Autodesk Fusion 360 part; units mm, degrees
(part 9 of 9)
  spline S33 degree 5 poles (15.6903, -6.8774) (15.6984, -6.8822) (15.7144, -6.892) (15.7381, -6.9074) (15.7688, -6.9292) (15.8062, -6.9579) (15.8428, -6.9878) (15.8789, -7.0185) (15.9148, -7.0495) (15.9505, -7.0809) (15.986, -7.1125) (16.0213, -7.1444) (16.0562, -7.1769) (16.0907, -7.2099) (16.1249, -7.2435) (16.1586, -7.2775) (16.1921, -7.3121) (16.2253, -7.3469) (16.2582, -7.3822) (16.2909, -7.4177) (16.3234, -7.4535) (16.3557, -7.4896) (16.3877, -7.526) (16.4194, -7.5628) (16.4509, -7.6) (16.4821, -7.6374) (16.5131, -7.6752) (16.5439, -7.7132) (16.5744, -7.7515) (16.6048, -7.7901) (16.6349, -7.829) (16.6647, -7.8681) (16.6944, -7.9075) (16.7238, -7.9471) (16.7531, -7.987) (16.7821, -8.0272) (16.8109, -8.0676) (16.8394, -8.1083) (16.8678, -8.1492) (16.896, -8.1903) (16.9239, -8.2317) (16.9517, -8.2733) (16.9792, -8.3151) (17.0066, -8.3572) (17.0337, -8.3994) (17.0607, -8.4419) (17.0874, -8.4846) (17.1139, -8.5276) (17.1403, -8.5707) (17.1664, -8.614) (17.1923, -8.6576) (17.2181, -8.7014) (17.2436, -8.7453) (17.269, -8.7895) (17.2941, -8.8338) (17.3191, -8.8784) (17.3438, -8.9231) (17.3684, -8.9681) (17.3928, -9.0132) (17.417, -9.0585) (17.441, -9.104) (17.4648, -9.1497) (17.4884, -9.1956) (17.5118, -9.2417) (17.535, -9.2879) (17.5581, -9.3343) (17.5809, -9.3809) (17.6036, -9.4277) (17.626, -9.4746) (17.6483, -9.5217) (17.6704, -9.569) (17.6879, -9.6069) (17.701, -9.6355) (17.7096, -9.6545) (17.7139, -9.6641) knots 0 0 0 0 0 0 0.01428571 0.02857143 0.04285714 0.05714286 0.07142857 0.08571429 0.1 0.11428571 0.12857143 0.14285714 0.15714286 0.17142857 0.18571429 0.2 0.21428571 0.22857143 0.24285714 0.25714286 0.27142857 0.28571429 0.3 0.31428571 0.32857143 0.34285714 0.35714286 0.37142857 0.38571429 0.4 0.41428571 0.42857143 0.44285714 0.45714286 0.47142857 0.48571429 0.5 0.51428571 0.52857143 0.54285714 0.55714286 0.57142857 0.58571429 0.6 0.61428571 0.62857143 0.64285714 0.65714286 0.67142857 0.68571429 0.7 0.71428571 0.72857143 0.74285714 0.75714286 0.77142857 0.78571429 0.8 0.81428571 0.82857143 0.84285714 0.85714286 0.87142857 0.88571429 0.9 0.91428571 0.92857143 0.94285714 0.95714286 0.97142857 0.98571429 1 1 1 1 1 1
  line L33 (15.6903, -6.8774) -> (15.3748, -6.6893)
  arc A67 (15.0406, -5.4943) -> (15.3748, -6.6893) centre (15.8355, -5.9162) ccw
  arc A68 (15.0406, -5.4943) -> (15.3066, -4.9723) centre (-0.4607, 2.7328) ccw
  arc A69 (16.4698, -4.5402) -> (15.3066, -4.9723) centre (16.1152, -5.3674) ccw
  line L34 (16.4698, -4.5402) -> (16.8074, -4.6849)
  spline S34 degree 5 poles (16.8074, -4.6849) (16.816, -4.6886) (16.8334, -4.6958) (16.8598, -4.7059) (16.8955, -4.7181) (16.9407, -4.7314) (16.9864, -4.7434) (17.0324, -4.7546) (17.0786, -4.7654) (17.125, -4.7759) (17.1714, -4.786) (17.218, -4.7957) (17.2648, -4.8049) (17.3118, -4.8135) (17.359, -4.8213) (17.4064, -4.8286) (17.454, -4.8354) (17.5017, -4.8417) (17.5496, -4.8477) (17.5975, -4.8533) (17.6456, -4.8585) (17.6938, -4.8634) (17.7421, -4.8679) (17.7905, -4.8719) (17.8391, -4.8756) (17.8877, -4.8788) (17.9365, -4.8817) (17.9853, -4.8842) (18.0343, -4.8864) (18.0833, -4.8883) (18.1325, -4.8898) (18.1817, -4.891) (18.231, -4.8918) (18.2803, -4.8923) (18.3298, -4.8925) (18.3794, -4.8924) (18.429, -4.8919) (18.4787, -4.8911) (18.5284, -4.89) (18.5783, -4.8886) (18.6282, -4.887) (18.6781, -4.885) (18.7282, -4.8827) (18.7782, -4.8801) (18.8284, -4.8772) (18.8786, -4.874) (18.9289, -4.8705) (18.9792, -4.8667) (19.0296, -4.8627) (19.08, -4.8584) (19.1305, -4.8537) (19.181, -4.8488) (19.2316, -4.8437) (19.2822, -4.8382) (19.3329, -4.8325) (19.3836, -4.8265) (19.4344, -4.8202) (19.4852, -4.8137) (19.536, -4.8069) (19.5869, -4.7998) (19.6378, -4.7925) (19.6888, -4.7849) (19.7398, -4.777) (19.7908, -4.7689) (19.8418, -4.7605) (19.8929, -4.7519) (19.944, -4.743) (19.9952, -4.7338) (20.0464, -4.7244) (20.0976, -4.7147) (20.1488, -4.7048) (20.1898, -4.6967) (20.2206, -4.6904) (20.2411, -4.6863) (20.2513, -4.6841) knots 0 0 0 0 0 0 0.01428571 0.02857143 0.04285714 0.05714286 0.07142857 0.08571429 0.1 0.11428571 0.12857143 0.14285714 0.15714286 0.17142857 0.18571429 0.2 0.21428571 0.22857143 0.24285714 0.25714286 0.27142857 0.28571429 0.3 0.31428571 0.32857143 0.34285714 0.35714286 0.37142857 0.38571429 0.4 0.41428571 0.42857143 0.44285714 0.45714286 0.47142857 0.48571429 0.5 0.51428571 0.52857143 0.54285714 0.55714286 0.57142857 0.58571429 0.6 0.61428571 0.62857143 0.64285714 0.65714286 0.67142857 0.68571429 0.7 0.71428571 0.72857143 0.74285714 0.75714286 0.77142857 0.78571429 0.8 0.81428571 0.82857143 0.84285714 0.85714286 0.87142857 0.88571429 0.9 0.91428571 0.92857143 0.94285714 0.95714286 0.97142857 0.98571429 1 1 1 1 1 1
  arc A70 (20.2513, -4.6841) -> (20.6552, -3.441) centre (-0.4607, 2.7328) ccw
  spline S35 degree 5 poles (17.8695, -1.4161) (17.8787, -1.4182) (17.897, -1.4226) (17.9242, -1.4299) (17.9602, -1.4411) (18.0046, -1.4569) (18.0487, -1.474) (18.0925, -1.492) (18.1362, -1.5104) (18.1799, -1.5292) (18.2234, -1.5483) (18.2668, -1.5678) (18.3101, -1.5879) (18.3531, -1.6086) (18.3959, -1.63) (18.4386, -1.6519) (18.4811, -1.6744) (18.5234, -1.6974) (18.5656, -1.7207) (18.6077, -1.7443) (18.6497, -1.7683) (18.6915, -1.7927) (18.7332, -1.8175) (18.7748, -1.8427) (18.8162, -1.8683) (18.8575, -1.8942) (18.8986, -1.9206) (18.9396, -1.9472) (18.9805, -1.9742) (19.0213, -2.0016) (19.0619, -2.0292) (19.1024, -2.0572) (19.1428, -2.0855) (19.183, -2.1141) (19.2232, -2.143) (19.2632, -2.1723) (19.303, -2.2018) (19.3428, -2.2316) (19.3824, -2.2618) (19.4219, -2.2922) (19.4613, -2.3229) (19.5005, -2.3539) (19.5397, -2.3851) (19.5786, -2.4167) (19.6175, -2.4485) (19.6563, -2.4806) (19.6949, -2.513) (19.7334, -2.5456) (19.7718, -2.5785) (19.81, -2.6116) (19.8482, -2.645) (19.8862, -2.6787) (19.924, -2.7126) (19.9618, -2.7468) (19.9994, -2.7812) (20.0369, -2.8158) (20.0743, -2.8507) (20.1116, -2.8859) (20.1487, -2.9213) (20.1857, -2.9569) (20.2226, -2.9928) (20.2593, -3.0289) (20.296, -3.0652) (20.3325, -3.1018) (20.3688, -3.1386) (20.4051, -3.1756) (20.4412, -3.2128) (20.4772, -3.2503) (20.5131, -3.288) (20.5488, -3.3259) (20.5844, -3.3641) (20.6128, -3.3947) (20.6341, -3.4179) (20.6482, -3.4333) (20.6552, -3.441) knots 0 0 0 0 0 0 0.01428571 0.02857143 0.04285714 0.05714286 0.07142857 0.08571429 0.1 0.11428571 0.12857143 0.14285714 0.15714286 0.17142857 0.18571429 0.2 0.21428571 0.22857143 0.24285714 0.25714286 0.27142857 0.28571429 0.3 0.31428571 0.32857143 0.34285714 0.35714286 0.37142857 0.38571429 0.4 0.41428571 0.42857143 0.44285714 0.45714286 0.47142857 0.48571429 0.5 0.51428571 0.52857143 0.54285714 0.55714286 0.57142857 0.58571429 0.6 0.61428571 0.62857143 0.64285714 0.65714286 0.67142857 0.68571429 0.7 0.71428571 0.72857143 0.74285714 0.75714286 0.77142857 0.78571429 0.8 0.81428571 0.82857143 0.84285714 0.85714286 0.87142857 0.88571429 0.9 0.91428571 0.92857143 0.94285714 0.95714286 0.97142857 0.98571429 1 1 1 1 1 1
  line L35 (17.8695, -1.4161) -> (17.5113, -1.3347)
  arc A71 (16.8242, -0.3015) -> (17.5113, -1.3347) centre (17.7106, -0.4571) ccw
  arc A72 (16.8242, -0.3015) -> (16.9158, 0.2772) centre (-0.4607, 2.7328) ccw
  arc A73 (17.8886, 1.0476) -> (16.9158, 0.2772) centre (17.807, 0.1513) ccw
  line L36 (17.8886, 1.0476) -> (18.2544, 1.0142)
  spline S36 degree 5 poles (18.2544, 1.0142) (18.2638, 1.0134) (18.2826, 1.0119) (18.3108, 1.0105) (18.3484, 1.01) (18.3956, 1.0112) (18.4427, 1.0139) (18.49, 1.0175) (18.5373, 1.0215) (18.5845, 1.0259) (18.6318, 1.0306) (18.6792, 1.0358) (18.7265, 1.0415) (18.7738, 1.0479) (18.8212, 1.055) (18.8685, 1.0627) (18.9159, 1.071) (18.9632, 1.0797) (19.0106, 1.0888) (19.0579, 1.0983) (19.1053, 1.1082) (19.1526, 1.1184) (19.1999, 1.1291) (19.2472, 1.1402) (19.2945, 1.1517) (19.3418, 1.1637) (19.3891, 1.176) (19.4363, 1.1887) (19.4835, 1.2018) (19.5307, 1.2152) (19.5779, 1.2289) (19.6251, 1.243) (19.6723, 1.2574) (19.7194, 1.2722) (19.7665, 1.2873) (19.8136, 1.3027) (19.8606, 1.3185) (19.9076, 1.3346) (19.9546, 1.351) (20.0016, 1.3677) (20.0485, 1.3848) (20.0954, 1.4021) (20.1423, 1.4198) (20.1891, 1.4377) (20.2359, 1.456) (20.2827, 1.4745) (20.3294, 1.4933) (20.3761, 1.5125) (20.4228, 1.5319) (20.4694, 1.5516) (20.516, 1.5716) (20.5625, 1.5919) (20.6091, 1.6124) (20.6555, 1.6332) (20.7019, 1.6543) (20.7483, 1.6757) (20.7947, 1.6974) (20.841, 1.7193) (20.8872, 1.7415) (20.9334, 1.7639) (20.9796, 1.7866) (21.0257, 1.8096) (21.0717, 1.8328) (21.1177, 1.8563) (21.1637, 1.8801) (21.2096, 1.9041) (21.2555, 1.9284) (21.3013, 1.9529) (21.3471, 1.9776) (21.3928, 2.0026) (21.4384, 2.0279) (21.4749, 2.0483) (21.5023, 2.0637) (21.5205, 2.0741) (21.5296, 2.0792) knots 0 0 0 0 0 0 0.01428571 0.02857143 0.04285714 0.05714286 0.07142857 0.08571429 0.1 0.11428571 0.12857143 0.14285714 0.15714286 0.17142857 0.18571429 0.2 0.21428571 0.22857143 0.24285714 0.25714286 0.27142857 0.28571429 0.3 0.31428571 0.32857143 0.34285714 0.35714286 0.37142857 0.38571429 0.4 0.41428571 0.42857143 0.44285714 0.45714286 0.47142857 0.48571429 0.5 0.51428571 0.52857143 0.54285714 0.55714286 0.57142857 0.58571429 0.6 0.61428571 0.62857143 0.64285714 0.65714286 0.67142857 0.68571429 0.7 0.71428571 0.72857143 0.74285714 0.75714286 0.77142857 0.78571429 0.8 0.81428571 0.82857143 0.84285714 0.85714286 0.87142857 0.88571429 0.9 0.91428571 0.92857143 0.94285714 0.95714286 0.97142857 0.98571429 1 1 1 1 1 1
  arc A74 (21.5296, 2.0792) -> (21.5296, 3.3863) centre (-0.4607, 2.7328) ccw
  spline S37 degree 5 poles (18.2544, 4.4513) (18.2638, 4.4522) (18.2826, 4.4536) (18.3108, 4.4551) (18.3484, 4.4556) (18.3956, 4.4543) (18.4427, 4.4516) (18.49, 4.4481) (18.5373, 4.444) (18.5845, 4.4396) (18.6318, 4.4349) (18.6792, 4.4298) (18.7265, 4.4241) (18.7738, 4.4177) (18.8212, 4.4106) (18.8685, 4.4029) (18.9159, 4.3946) (18.9632, 4.3859) (19.0106, 4.3768) (19.0579, 4.3673) (19.1053, 4.3574) (19.1526, 4.3471) (19.1999, 4.3365) (19.2472, 4.3253) (19.2945, 4.3138) (19.3418, 4.3019) (19.3891, 4.2895) (19.4363, 4.2769) (19.4835, 4.2638) (19.5307, 4.2504) (19.5779, 4.2367) (19.6251, 4.2226) (19.6723, 4.2082) (19.7194, 4.1934) (19.7665, 4.1783) (19.8136, 4.1628) (19.8606, 4.1471) (19.9076, 4.131) (19.9546, 4.1145) (20.0016, 4.0978) (20.0485, 4.0808) (20.0954, 4.0634) (20.1423, 4.0458) (20.1891, 4.0279) (20.2359, 4.0096) (20.2827, 3.9911) (20.3294, 3.9722) (20.3761, 3.9531) (20.4228, 3.9337) (20.4694, 3.914) (20.516, 3.894) (20.5625, 3.8737) (20.6091, 3.8532) (20.6555, 3.8323) (20.7019, 3.8112) (20.7483, 3.7898) (20.7947, 3.7682) (20.841, 3.7463) (20.8872, 3.7241) (20.9334, 3.7016) (20.9796, 3.6789) (21.0257, 3.656) (21.0717, 3.6327) (21.1177, 3.6092) (21.1637, 3.5855) (21.2096, 3.5615) (21.2555, 3.5372) (21.3013, 3.5127) (21.3471, 3.4879) (21.3928, 3.4629) (21.4384, 3.4376) (21.4749, 3.4172) (21.5023, 3.4018) (21.5205, 3.3915) (21.5296, 3.3863) knots 0 0 0 0 0 0 0.01428571 0.02857143 0.04285714 0.05714286 0.07142857 0.08571429 0.1 0.11428571 0.12857143 0.14285714 0.15714286 0.17142857 0.18571429 0.2 0.21428571 0.22857143 0.24285714 0.25714286 0.27142857 0.28571429 0.3 0.31428571 0.32857143 0.34285714 0.35714286 0.37142857 0.38571429 0.4 0.41428571 0.42857143 0.44285714 0.45714286 0.47142857 0.48571429 0.5 0.51428571 0.52857143 0.54285714 0.55714286 0.57142857 0.58571429 0.6 0.61428571 0.62857143 0.64285714 0.65714286 0.67142857 0.68571429 0.7 0.71428571 0.72857143 0.74285714 0.75714286 0.77142857 0.78571429 0.8 0.81428571 0.82857143 0.84285714 0.85714286 0.87142857 0.88571429 0.9 0.91428571 0.92857143 0.94285714 0.95714286 0.97142857 0.98571429 1 1 1 1 1 1
  line L37 (18.2544, 4.4513) -> (17.8886, 4.418)
  arc A75 (16.9158, 5.1884) -> (17.8886, 4.418) centre (17.807, 5.3143) ccw
  arc A76 (16.9158, 5.1884) -> (16.8242, 5.767) centre (-0.4607, 2.7328) ccw
  arc A77 (17.5113, 6.8003) -> (16.8242, 5.767) centre (17.7106, 5.9227) ccw
  line L38 (17.5113, 6.8003) -> (17.8695, 6.8816)
  spline S38 degree 5 poles (17.8695, 6.8816) (17.8787, 6.8837) (17.897, 6.8881) (17.9242, 6.8955) (17.9602, 6.9066) (18.0046, 6.9224) (18.0487, 6.9396) (18.0925, 6.9575) (18.1362, 6.976) (18.1799, 6.9948) (18.2234, 7.0138) (18.2668, 7.0334) (18.3101, 7.0534) (18.3531, 7.0742) (18.3959, 7.0955) (18.4386, 7.1175) (18.4811, 7.14) (18.5234, 7.1629) (18.5656, 7.1862) (18.6077, 7.2099) (18.6497, 7.2339) (18.6915, 7.2583) (18.7332, 7.2831) (18.7748, 7.3082) (18.8162, 7.3338) (18.8575, 7.3598) (18.8986, 7.3861) (18.9396, 7.4128) (18.9805, 7.4398) (19.0213, 7.4671) (19.0619, 7.4948) (19.1024, 7.5228) (19.1428, 7.551) (19.183, 7.5797) (19.2232, 7.6086) (19.2632, 7.6378) (19.303, 7.6674) (19.3428, 7.6972) (19.3824, 7.7273) (19.4219, 7.7577) (19.4613, 7.7884) (19.5005, 7.8194) (19.5397, 7.8507) (19.5786, 7.8822) (19.6175, 7.9141) (19.6563, 7.9462) (19.6949, 7.9785) (19.7334, 8.0111) (19.7718, 8.044) (19.81, 8.0772) (19.8482, 8.1106) (19.8862, 8.1442) (19.924, 8.1782) (19.9618, 8.2123) (19.9994, 8.2467) (20.0369, 8.2814) (20.0743, 8.3163) (20.1116, 8.3515) (20.1487, 8.3868) (20.1857, 8.4225) (20.2226, 8.4583) (20.2593, 8.4944) (20.296, 8.5308) (20.3325, 8.5673) (20.3688, 8.6041) (20.4051, 8.6412) (20.4412, 8.6784) (20.4772, 8.7159) (20.5131, 8.7536) (20.5488, 8.7915) (20.5844, 8.8296) (20.6128, 8.8603) (20.6341, 8.8834) (20.6482, 8.8989) (20.6552, 8.9066) knots 0 0 0 0 0 0 0.01428571 0.02857143 0.04285714 0.05714286 0.07142857 0.08571429 0.1 0.11428571 0.12857143 0.14285714 0.15714286 0.17142857 0.18571429 0.2 0.21428571 0.22857143 0.24285714 0.25714286 0.27142857 0.28571429 0.3 0.31428571 0.32857143 0.34285714 0.35714286 0.37142857 0.38571429 0.4 0.41428571 0.42857143 0.44285714 0.45714286 0.47142857 0.48571429 0.5 0.51428571 0.52857143 0.54285714 0.55714286 0.57142857 0.58571429 0.6 0.61428571 0.62857143 0.64285714 0.65714286 0.67142857 0.68571429 0.7 0.71428571 0.72857143 0.74285714 0.75714286 0.77142857 0.78571429 0.8 0.81428571 0.82857143 0.84285714 0.85714286 0.87142857 0.88571429 0.9 0.91428571 0.92857143 0.94285714 0.95714286 0.97142857 0.98571429 1 1 1 1 1 1
  arc A78 (20.6552, 8.9066) -> (20.2513, 10.1497) centre (-0.4607, 2.7328) ccw
  spline S39 degree 5 poles (16.8074, 10.1505) (16.816, 10.1542) (16.8334, 10.1614) (16.8598, 10.1715) (16.8955, 10.1836) (16.9407, 10.197) (16.9864, 10.209) (17.0324, 10.2202) (17.0786, 10.231) (17.125, 10.2414) (17.1714, 10.2516) (17.218, 10.2613) (17.2648, 10.2705) (17.3118, 10.279) (17.359, 10.2869) (17.4064, 10.2942) (17.454, 10.301) (17.5017, 10.3073) (17.5496, 10.3133) (17.5975, 10.3189) (17.6456, 10.3241) (17.6938, 10.329) (17.7421, 10.3334) (17.7905, 10.3375) (17.8391, 10.3411) (17.8877, 10.3444) (17.9365, 10.3473) (17.9853, 10.3498) (18.0343, 10.352) (18.0833, 10.3538) (18.1325, 10.3553) (18.1817, 10.3565) (18.231, 10.3574) (18.2803, 10.3579) (18.3298, 10.3581) (18.3794, 10.3579) (18.429, 10.3575) (18.4787, 10.3567) (18.5284, 10.3556) (18.5783, 10.3542) (18.6282, 10.3525) (18.6781, 10.3505) (18.7282, 10.3482) (18.7782, 10.3456) (18.8284, 10.3427) (18.8786, 10.3395) (18.9289, 10.3361) (18.9792, 10.3323) (19.0296, 10.3282) (19.08, 10.3239) (19.1305, 10.3193) (19.181, 10.3144) (19.2316, 10.3092) (19.2822, 10.3038) (19.3329, 10.2981) (19.3836, 10.2921) (19.4344, 10.2858) (19.4852, 10.2793) (19.536, 10.2724) (19.5869, 10.2654) (19.6378, 10.258) (19.6888, 10.2504) (19.7398, 10.2426) (19.7908, 10.2344) (19.8418, 10.2261) (19.8929, 10.2174) (19.944, 10.2085) (19.9952, 10.1994) (20.0464, 10.1899) (20.0976, 10.1803) (20.1488, 10.1704) (20.1898, 10.1622) (20.2206, 10.156) (20.2411, 10.1518) (20.2513, 10.1497) knots 0 0 0 0 0 0 0.01428571 0.02857143 0.04285714 0.05714286 0.07142857 0.08571429 0.1 0.11428571 0.12857143 0.14285714 0.15714286 0.17142857 0.18571429 0.2 0.21428571 0.22857143 0.24285714 0.25714286 0.27142857 0.28571429 0.3 0.31428571 0.32857143 0.34285714 0.35714286 0.37142857 0.38571429 0.4 0.41428571 0.42857143 0.44285714 0.45714286 0.47142857 0.48571429 0.5 0.51428571 0.52857143 0.54285714 0.55714286 0.57142857 0.58571429 0.6 0.61428571 0.62857143 0.64285714 0.65714286 0.67142857 0.68571429 0.7 0.71428571 0.72857143 0.74285714 0.75714286 0.77142857 0.78571429 0.8 0.81428571 0.82857143 0.84285714 0.85714286 0.87142857 0.88571429 0.9 0.91428571 0.92857143 0.94285714 0.95714286 0.97142857 0.98571429 1 1 1 1 1 1
  line L39 (16.8074, 10.1505) -> (16.4698, 10.0058)
  arc A79 (15.3066, 10.4378) -> (16.4698, 10.0058) centre (16.1152, 10.833) ccw
  arc A80 (15.3066, 10.4378) -> (15.0406, 10.9599) centre (-0.4607, 2.7328) ccw
  circle A81 centre (-0.4607, 2.7328) radius 15
  constraint concentric A0 A81
extrude "Extrude3'''" add sketch "Sketch7" along normal blind 3 contours A0 A81 | A1 L0 S0 A2 S1 L1 A3 A4 A5 L2 S2 A6 S3 L3 A7 A8 A9 L4 S4 A10 S5 L5 A11 A12 A13 L6 S6 A14 S7 L7 A15 A16 A17 L8 S8 A18 S9 L9 A19 A20 A21 L10 S10 A22 S11 L11 A23 A24 A25 L12 S12 A26 S13 L13 A27 A28 A29 L14 S14 A30 S15 L15 A31 A32 A33 L16 S16 A34 S17 L17 A35 A36 A37 L18 S18 A38 S19 L19 A39 A40 A41 L20 S20 A42 S21 L21 A43 A44 A45 L22 S22 A46 S23 L23 A47 A48 A49 L24 S24 A50 S25 L25 A51 A52 A53 L26 S26 A54 S27 L27 A55 A56 A57 L28 S28 A58 S29 L29 A59 A60 A61 L30 S30 A62 S31 L31 A63 A64 A65 L32 S32 A66 S33 L33 A67 A68 A69 L34 S34 A70 S35 L35 A71 A72 A73 L36 S36 A74 S37 L37 A75 A76 A77 L38 S38 A78 S39 L39 A79 A80 sketch seen with x (1, 0, 0) y (0, 1, 0) z (0, 0, 1) at (0.4607, 2.7328, 0.7135) bodies 1 in component "Spur Gear (20 teeth) (1)"
extrude "Extrude4" add 1 faces at (6.2724, -0.5, 0) along direction (0, 0, -1) blind 3 on bodies 3 bodies 3 in component "Spur Gear (11 teeth)"
extrude "Extrude4'" add 1 faces at (5.611, 0.4837, 0) along direction (0, 0, -1) blind 3 on bodies 4 bodies 4 in component "Spur Gear (10 teeth)"
extrude "Extrude6" add 1 faces at (2.8046, -0.4499, 0) along direction (0, 0, -1) blind 3 on bodies 5 bodies 5 in component "Spur Gear (7 teeth)"
component "Spur Gear (20 teeth) (1)" placed x (1, 0, 0) y (0, 1, 0) z (0, 0, 1) at (-0.4607, -2.7328, -0.7135)
component "Spur Gear (22 teeth)" placed x (1, 0, 0) y (0, 1, 0) z (0, 0, 1) at (48.0648, -1.0985, -0.2907)
component "Spur Gear (11 teeth)" placed x (1, 0, 0) y (0, 1, 0) z (0, 0, 1) at (44.9504, 37.7771, -0.209)
component "Spur Gear (10 teeth)" placed x (1, 0, 0) y (0, 1, 0) z (0, 0, 1) at (19.0845, 30.7575, -1.2301)
component "Spur Gear (7 teeth)" placed x (1, 0, 0) y (0, 1, 0) z (0, 0, 1) at (-5.086, 30.7162, -0.1053)
